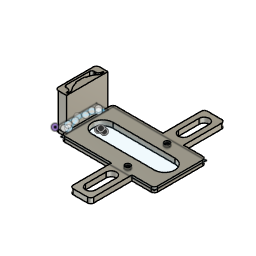
daq_cclamp_3b (v3~recovered) (Autodesk Fusion 360 design; units mm, degrees)
Autodesk Fusion 360 part; units mm, degrees
note: some values were not read from the file. Set by a fixed rule: which sketch regions a step uses.
sketch "Sketch1" plane through (0, 0, 0) normal (0, 0, 1) x (1, 0, 0)
  line L0 (0, 0) -> (11, 0)
  line L1 (11, 0) -> (11, 40)
  line L2 (11, 40) -> (0, 40)
  line L3 (0, 40) -> (0, 0)
  line L4 (2, 31.5) -> (2, 8.5)
  line L5 (8.5, 2.5) -> (9.5, 2.5)
  arc A0 (4.9716, 15.1064) -> (4.4831, 15.5) centre (4.4831, 15) ccw
  arc A1 (9.5, 5.5) -> (9.021, 6.7987) centre (7.5, 5.5) ccw
  line L6 (9.5, 34.5) -> (9.5, 37.5)
  arc A2 (8.5, 3.5) -> (5.5, 6.5) centre (5.5, 3.5) ccw
  arc A3 (5.7416, 27.6132) -> (5.6837, 27.4547) centre (23.0901, 21.1884) ccw
  arc A4 (5.7416, 12.3868) -> (5.8046, 12.2095) centre (27.445, 20) ccw
  line L7 (5.6837, 27.4547) -> (5.8046, 27.7905)
  arc A5 (5.7416, 12.3868) -> (9.021, 6.7987) centre (23.0901, 18.8116) ccw
  arc A6 (5.7416, 27.6132) -> (4.9716, 24.8936) centre (27.445, 20) ccw
  arc A7 (4, 33.5) -> (2, 31.5) centre (4, 31.5) ccw
  line L8 (9.5, 37.5) -> (8.5, 37.5)
  line L9 (4.1215, 24.5) -> (4.4831, 24.5)
  arc A8 (2, 8.5) -> (4, 6.5) centre (4, 8.5) ccw
  arc A9 (5.5, 33.5) -> (8.5, 36.5) centre (5.5, 36.5) ccw
  line L10 (5.5, 33.5) -> (4, 33.5)
  line L11 (4, 6.5) -> (5.5, 6.5)
  line L12 (9.5, 2.5) -> (9.5, 5.5)
  line L13 (8.5, 37.5) -> (8.5, 36.5)
  line L14 (4.4831, 15.5) -> (4.1215, 15.5)
  arc A10 (9.021, 33.2013) -> (5.7416, 27.6132) centre (23.0901, 21.1884) ccw
  arc A11 (9.021, 33.2013) -> (9.5, 34.5) centre (7.5, 34.5) ccw
  line L15 (5.8046, 12.2095) -> (5.6837, 12.5453)
  line L16 (8.5, 3.5) -> (8.5, 2.5)
  arc A12 (5.8046, 27.7905) -> (5.7416, 27.6132) centre (27.445, 20) ccw
  arc A13 (5.6837, 12.5453) -> (5.7416, 12.3868) centre (23.0901, 18.8116) ccw
  line L17 (4.1215, 15.5) -> (4.1215, 24.5)
  arc A14 (4.9716, 15.1064) -> (5.7416, 12.3868) centre (27.445, 20) ccw
  arc A15 (4.4831, 24.5) -> (4.9716, 24.8936) centre (4.4831, 25) ccw
  line L18 (11, 45) -> (101, 45)
  line L19 (101, 45) -> (101, -5)
  line L20 (101, -5) -> (11, -5)
  line L21 (11, -5) -> (11, 45)
  circle A16 centre (69.31, 39.05) radius 2.5
  circle A17 centre (69.31, 0.95) radius 2.5
  arc A18 (9.097, 33.1364) -> (5.8357, 27.5793) centre (23.0901, 21.1884) ccw
  arc A19 (5.8357, 27.5793) -> (5.0693, 24.8723) centre (27.445, 20) ccw
  arc A20 (4.4831, 24.4) -> (5.0693, 24.8723) centre (4.4831, 25) ccw
  line L22 (4.2215, 24.4) -> (4.4831, 24.4)
  line L23 (4.2215, 15.6) -> (4.2215, 24.4)
  line L24 (4.4831, 15.6) -> (4.2215, 15.6)
  arc A21 (5.0693, 15.1277) -> (4.4831, 15.6) centre (4.4831, 15) ccw
  arc A22 (5.0693, 15.1277) -> (5.8357, 12.4207) centre (27.445, 20) ccw
  arc A23 (5.8357, 12.4207) -> (9.097, 6.8636) centre (23.0901, 18.8116) ccw
  arc A24 (9.6, 5.5) -> (9.097, 6.8636) centre (7.5, 5.5) ccw
  line L25 (9.6, 2.4) -> (9.6, 5.5)
  line L26 (8.4, 2.4) -> (9.6, 2.4)
  line L27 (8.4, 3.5) -> (8.4, 2.4)
  arc A25 (8.4, 3.5) -> (5.5, 6.4) centre (5.5, 3.5) ccw
  line L28 (4, 6.4) -> (5.5, 6.4)
  arc A26 (1.9, 8.5) -> (4, 6.4) centre (4, 8.5) ccw
  line L29 (1.9, 31.5) -> (1.9, 8.5)
  arc A27 (4, 33.6) -> (1.9, 31.5) centre (4, 31.5) ccw
  line L30 (5.5, 33.6) -> (4, 33.6)
  arc A28 (5.5, 33.6) -> (8.4, 36.5) centre (5.5, 36.5) ccw
  line L31 (8.4, 37.6) -> (8.4, 36.5)
  line L32 (9.6, 37.6) -> (8.4, 37.6)
  line L33 (9.6, 34.5) -> (9.6, 37.6)
  arc A29 (9.097, 33.1364) -> (9.6, 34.5) centre (7.5, 34.5) ccw
  point P0 (1.7277, 20)
  dimension "d1" = 11
  dimension "d2" = 40
  dimension "d3" = 90
  dimension "d4" = 50
  dimension "d5" = 5
  dimension "d6" = 5
  dimension "d7" = 58.31
  dimension "d8" = 58.31
  dimension "d9" = 38.1
  dimension "d10" = 5.95
  dimension "d56" = 0.1
  constraint horizontal L0
  constraint vertical L1
  constraint horizontal L2
  constraint vertical L3
  constraint coincident L0.start L3.end
  constraint horizontal L18
  constraint vertical L19
  constraint horizontal L20
  constraint vertical L21
  constraint midpoint L1 L21
  measures "d1" distance of L0.start L0.end
  measures "d2" distance of L0.start L2.end
  measures "d3" distance of L18.start L18.end
  measures "d4" distance of L18.start L20.end
  measures "d5" diameter of A16
  measures "d6" diameter of A17
  measures "d7" distance of L21 A16.centre
  measures "d8" distance of L1 A17.centre
  measures "d9" distance of A16.centre A17.centre
  measures "d10" distance of L18 A16.centre
extrude "Extrude1" add sketch "Sketch1" along normal blind 2 contours L0 L1 L2 L3 L21 | L1 L18 L19 L20 L21
fillet "Fillet1" radius 3 6 edges at (101, -5, 1) (101, 45, 1) (11, -5, 1) (0, 0, 1) (11, 45, 1) (0, 40, 1)
sketch "Sketch2" plane through (0, 0, 2) normal (0, 0, 1) x (-1, 0, 0)
  arc A0 (-3, -40) -> (0, -37) centre (-3, -37) ccw
  line L0 (0, -37) -> (0, -3)
  arc A1 (0, -3) -> (-3, 0) centre (-3, -3) ccw
  line L1 (-3, 0) -> (-11, 0)
  line L2 (-11, 0) -> (-11, 2)
  arc A2 (-11, 2) -> (-14, 5) centre (-14, 2) ccw
  line L3 (-14, 5) -> (-98, 5)
  arc A3 (-98, 5) -> (-101, 2) centre (-98, 2) ccw
  line L4 (-101, 2) -> (-101, -42)
  arc A4 (-101, -42) -> (-98, -45) centre (-98, -42) ccw
  line L5 (-98, -45) -> (-14, -45)
  arc A5 (-14, -45) -> (-11, -42) centre (-14, -42) ccw
  line L6 (-11, -42) -> (-11, -40)
  line L7 (-11, -40) -> (-3, -40)
  circle A6 centre (-69.31, -0.95) radius 2.5
  circle A7 centre (-69.31, -39.05) radius 2.5
  line L8 (-11, -40) -> (-11, 0)
  arc A8 (-9.097, -33.1364) -> (-5.8357, -27.5793) centre (-23.0901, -21.1884) ccw
  arc A9 (-5.8357, -27.5793) -> (-5.0693, -24.8723) centre (-27.445, -20) ccw
  arc A10 (-4.4831, -24.4) -> (-5.0693, -24.8723) centre (-4.4831, -25) ccw
  line L9 (-4.4831, -24.4) -> (-4.2215, -24.4)
  line L10 (-4.2215, -24.4) -> (-4.2215, -15.6)
  line L11 (-4.2215, -15.6) -> (-4.4831, -15.6)
  arc A11 (-5.0693, -15.1277) -> (-4.4831, -15.6) centre (-4.4831, -15) ccw
  arc A12 (-5.0693, -15.1277) -> (-5.8357, -12.4207) centre (-27.445, -20) ccw
  arc A13 (-5.8357, -12.4207) -> (-9.097, -6.8636) centre (-23.0901, -18.8116) ccw
  arc A14 (-9.6, -5.5) -> (-9.097, -6.8636) centre (-7.5, -5.5) ccw
  line L12 (-9.6, -5.5) -> (-9.6, -2.4)
  line L13 (-9.6, -2.4) -> (-8.4, -2.4)
  line L14 (-8.4, -2.4) -> (-8.4, -3.5)
  arc A15 (-8.4, -3.5) -> (-5.5, -6.4) centre (-5.5, -3.5) ccw
  line L15 (-5.5, -6.4) -> (-4, -6.4)
  arc A16 (-1.9, -8.5) -> (-4, -6.4) centre (-4, -8.5) ccw
  line L16 (-1.9, -8.5) -> (-1.9, -31.5)
  arc A17 (-4, -33.6) -> (-1.9, -31.5) centre (-4, -31.5) ccw
  line L17 (-4, -33.6) -> (-5.5, -33.6)
  arc A18 (-5.5, -33.6) -> (-8.4, -36.5) centre (-5.5, -36.5) ccw
  line L18 (-8.4, -36.5) -> (-8.4, -37.6)
  line L19 (-8.4, -37.6) -> (-9.6, -37.6)
  line L20 (-9.6, -37.6) -> (-9.6, -34.5)
  arc A19 (-9.097, -33.1364) -> (-9.6, -34.5) centre (-7.5, -34.5) ccw
  constraint coincident L6.end L7.start
  constraint coincident L1.end L2.start
extrude "Extrude2" add sketch "Sketch2" along normal blind 30 and the other way blind 2 contours A0 L0 A1 L1 L7 L8
sketch "Sketch7" plane through (0, 0, 0) normal (0, 0, -1) x (1, 0, 0)
  circle A0 centre (69.31, -39.05) radius 2.5
  circle A1 centre (69.31, -0.95) radius 2.5
  arc A2 (0, -37) -> (3, -40) centre (3, -37) ccw
  line L0 (3, -40) -> (11, -40)
  line L1 (11, -40) -> (11, -42)
  arc A3 (11, -42) -> (14, -45) centre (14, -42) ccw
  line L2 (14, -45) -> (98, -45)
  arc A4 (98, -45) -> (101, -42) centre (98, -42) ccw
  line L3 (101, -42) -> (101, 2)
  arc A5 (101, 2) -> (98, 5) centre (98, 2) ccw
  line L4 (98, 5) -> (14, 5)
  arc A6 (14, 5) -> (11, 2) centre (14, 2) ccw
  line L5 (11, 2) -> (11, 0)
  line L6 (11, 0) -> (3, 0)
  arc A7 (3, 0) -> (0, -3) centre (3, -3) ccw
  line L7 (0, -3) -> (0, -37)
  circle A8 centre (69.31, -0.95) radius 4.5
  circle A9 centre (69.31, -39.05) radius 4.5
  arc A10 (5.8357, -27.5793) -> (9.097, -33.1364) centre (23.0901, -21.1884) ccw
  arc A11 (9.6, -34.5) -> (9.097, -33.1364) centre (7.5, -34.5) ccw
  line L8 (9.6, -34.5) -> (9.6, -37.6)
  line L9 (9.6, -37.6) -> (8.4, -37.6)
  line L10 (8.4, -37.6) -> (8.4, -36.5)
  arc A12 (8.4, -36.5) -> (5.5, -33.6) centre (5.5, -36.5) ccw
  line L11 (5.5, -33.6) -> (4, -33.6)
  arc A13 (1.9, -31.5) -> (4, -33.6) centre (4, -31.5) ccw
  line L12 (1.9, -31.5) -> (1.9, -8.5)
  arc A14 (4, -6.4) -> (1.9, -8.5) centre (4, -8.5) ccw
  line L13 (4, -6.4) -> (5.5, -6.4)
  arc A15 (5.5, -6.4) -> (8.4, -3.5) centre (5.5, -3.5) ccw
  line L14 (8.4, -3.5) -> (8.4, -2.4)
  line L15 (8.4, -2.4) -> (9.6, -2.4)
  line L16 (9.6, -2.4) -> (9.6, -5.5)
  arc A16 (9.097, -6.8636) -> (9.6, -5.5) centre (7.5, -5.5) ccw
  arc A17 (9.097, -6.8636) -> (5.8357, -12.4207) centre (23.0901, -18.8116) ccw
  arc A18 (5.8357, -12.4207) -> (5.0693, -15.1277) centre (27.445, -20) ccw
  arc A19 (4.4831, -15.6) -> (5.0693, -15.1277) centre (4.4831, -15) ccw
  line L17 (4.4831, -15.6) -> (4.2215, -15.6)
  line L18 (4.2215, -15.6) -> (4.2215, -24.4)
  line L19 (4.2215, -24.4) -> (4.4831, -24.4)
  arc A20 (5.0693, -24.8723) -> (4.4831, -24.4) centre (4.4831, -25) ccw
  arc A21 (5.0693, -24.8723) -> (5.8357, -27.5793) centre (27.445, -20) ccw
  dimension "d48" = 9
  dimension "d49" = 9
  constraint concentric A1 A8
  constraint concentric A0 A9
  measures "d48" diameter of A8
  measures "d49" diameter of A9
extrude "Extrude7" add sketch "Sketch7" along normal blind 3 contours A2 L0 L1 A3 L2 A4 L3 A5 L4 A6 L5 L6 A7 L7
sketch "Sketch10" plane through (0, 0, 2) normal (0, 0, 1) x (-1, 0, 0)
  line L0 (-11, -40) -> (-11, 0)
  line L1 (-11, 0) -> (-11, 2)
  arc A0 (-11, 2) -> (-14, 5) centre (-14, 2) ccw
  line L2 (-14, 5) -> (-98, 5)
  arc A1 (-98, 5) -> (-101, 2) centre (-98, 2) ccw
  line L3 (-101, 2) -> (-101, -42)
  arc A2 (-101, -42) -> (-98, -45) centre (-98, -42) ccw
  line L4 (-98, -45) -> (-14, -45)
  arc A3 (-14, -45) -> (-11, -42) centre (-14, -42) ccw
  line L5 (-11, -42) -> (-11, -40)
  circle A4 centre (-69.31, -0.95) radius 2.5
  circle A5 centre (-69.31, -39.05) radius 2.5
  line L6 (-59.31, -45) -> (-79.31, -45)
  line L7 (-79.31, -45) -> (-79.31, -82)
  line L8 (-76.31, -85) -> (-62.31, -85)
  line L9 (-59.31, -82) -> (-59.31, -45)
  line L10 (-69.31, -39.05) -> (-69.31, -85)
  arc A6 (-62.31, -85) -> (-59.31, -82) centre (-62.31, -82) ccw
  arc A7 (-79.31, -82) -> (-76.31, -85) centre (-76.31, -82) ccw
  line L11 (0, -20) -> (-101, -20)
  arc A8 (-76.31, 45) -> (-79.31, 42) centre (-76.31, 42) ccw
  line L12 (-59.31, 42) -> (-59.31, 5)
  line L13 (-59.31, 5) -> (-79.31, 5)
  line L14 (-76.31, 45) -> (-62.31, 45)
  arc A9 (-59.31, 42) -> (-62.31, 45) centre (-62.31, 42) ccw
  line L15 (-79.31, 5) -> (-79.31, 42)
  point P0 (-59.31, -85)
  point P1 (-59.31, 45)
  point P2 (-69.31, 45)
  dimension "d59" = 20
  dimension "d60" = 40
  dimension "d61" = 10
  dimension "d62" = 3
  constraint horizontal L6
  constraint vertical L7
  constraint horizontal L8
  constraint vertical L9
  constraint coincident L4 L6.start
  constraint coincident A5.centre L10.start
  constraint coincident L8 L10.end
  constraint perpendicular L8 L10
  constraint coincident P0 L8
  constraint coincident P0 L9
  constraint tangent L8 A6
  constraint tangent L9 A6
  constraint tangent L7 A7
  constraint tangent L8 A7
  constraint equal A6 A7
  constraint midpoint L3 L11.end
  constraint perpendicular L3 L11
  constraint symmetric L6.start L11 L12.end
  constraint symmetric L6.end L11 L13.end
  constraint symmetric P0 L11 P1
  constraint symmetric L10.end L11 P2
  constraint symmetric L8.end L11 L14.end
  constraint symmetric L9.start L11 L12.start
  constraint symmetric A6 L11 A9
  constraint symmetric L7.end L11 A8.end
  constraint symmetric L8.start L11 A8.start
  constraint symmetric A7 L11 A8
  measures "d59" distance of L6.start L6.end
  measures "d60" distance of L6.start P0
  measures "d61" distance of L7 L10
  measures "d62" radius of A6
extrude "Extrude9" add sketch "Sketch10" against normal blind 5 contours L4 L6 L8 L9 L10 A6 | L4 L6 L7 L8 L10 A7 | L2 A8 L12 L13 L14 A9 L15
sketch "Sketch11" plane through (0, 0, 2) normal (0, 0, 1) x (-1, 0, 0)
  line L0 (-11, -40) -> (-11, 0)
  line L1 (-11, 0) -> (-11, 2)
  arc A0 (-11, 2) -> (-14, 5) centre (-14, 2) ccw
  line L2 (-14, 5) -> (-59.31, 5)
  line L3 (-59.31, 5) -> (-59.31, 42)
  arc A1 (-59.31, 42) -> (-62.31, 45) centre (-62.31, 42) ccw
  line L4 (-62.31, 45) -> (-76.31, 45)
  arc A2 (-76.31, 45) -> (-79.31, 42) centre (-76.31, 42) ccw
  line L5 (-79.31, 42) -> (-79.31, 5)
  line L6 (-79.31, 5) -> (-98, 5)
  arc A3 (-98, 5) -> (-101, 2) centre (-98, 2) ccw
  line L7 (-101, 2) -> (-101, -42)
  arc A4 (-101, -42) -> (-98, -45) centre (-98, -42) ccw
  line L8 (-98, -45) -> (-79.31, -45)
  line L9 (-79.31, -45) -> (-79.31, -82)
  arc A5 (-79.31, -82) -> (-76.31, -85) centre (-76.31, -82) ccw
  line L10 (-76.31, -85) -> (-62.31, -85)
  arc A6 (-62.31, -85) -> (-59.31, -82) centre (-62.31, -82) ccw
  line L11 (-59.31, -82) -> (-59.31, -45)
  line L12 (-59.31, -45) -> (-14, -45)
  arc A7 (-14, -45) -> (-11, -42) centre (-14, -42) ccw
  line L13 (-11, -42) -> (-11, -40)
  circle A8 centre (-69.31, -0.95) radius 2.5
  circle A9 centre (-69.31, -39.05) radius 2.5
  line L14 (-59.31, 5) -> (-79.31, 5)
  line L15 (-59.31, -45) -> (-79.31, -45)
  line L16 (-64.31, 10) -> (-74.31, 10)
  line L17 (-74.31, 10) -> (-74.31, 40)
  line L18 (-74.31, 40) -> (-64.31, 40)
  line L19 (-64.31, 40) -> (-64.31, 10)
  line L20 (-64.31, -50) -> (-74.31, -50)
  line L21 (-74.31, -50) -> (-74.31, -80)
  line L22 (-64.31, -80) -> (-64.31, -50)
  line L23 (-74.31, -80) -> (-64.31, -80)
  line L24 (-16, -30) -> (-96, -30)
  line L25 (-96, -30) -> (-96, -10)
  line L26 (-96, -10) -> (-16, -10)
  line L27 (-16, -10) -> (-16, -30)
  dimension "d65" = 10
  dimension "d66" = 30
  dimension "d67" = 5
  dimension "d68" = 5
  dimension "d69" = 80
  dimension "d70" = 20
  dimension "d71" = 5
  constraint coincident L2.end L3.start
  constraint coincident L5.end L6.start
  constraint coincident L11.end L12.start
  constraint coincident L8.end L9.start
  constraint horizontal L16
  constraint vertical L17
  constraint horizontal L18
  constraint vertical L19
  constraint horizontal L24
  constraint vertical L25
  constraint horizontal L26
  constraint vertical L27
  measures "d65" distance of L16.start L16.end
  measures "d66" distance of L16.start L18.end
  measures "d67" distance of L5 L17
  measures "d68" distance of L14 L16
  measures "d69" distance of L24.start L24.end
  measures "d70" distance of L24.start L26.end
  measures "d71" distance of L7 L25
extrude "Extrude10" cut sketch "Sketch11" against normal blind 5 contours L16 L17 L18 L19 | L20 L21 L22 L23 | L24 L25 L26 L27
fillet "Fillet2" radius 10 4 edges at (16, 10, -0.5) (16, 30, -0.5) (96, 10, -0.5) (96, 30, -0.5)
fillet "Fillet3" radius 5 4 edges at (64.31, -10, -0.5) (74.31, -40, -0.5) (64.31, -40, -0.5) (74.31, -10, -0.5)
fillet "Fillet4" radius 5 4 edges at (64.31, 50, -0.5) (74.31, 50, -0.5) (64.31, 80, -0.5) (74.31, 80, -0.5)
